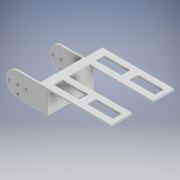
# Autodesk Inventor part: Claw
Saved by Autodesk Inventor 2020 (Build 240168000, 168)
## iProperties
Created: 2020-01-09
Part Number: Claw
Material: 일반
Document SubType Name: Modeling
Designer: Knowblesse
Density: 1 g/cm^3
Appearance: 기본값
Author: Knowblesse
Autodesk Inventor part; units mm, degrees
ref_plane "YZ Plane" through (0, 0, 0) normal (1, 0, 0) x (0, 1, 0)
ref_plane "XZ Plane" through (0, 0, 0) normal (0, 1, 0) x (-1, 0, 0)
ref_plane "XY Plane" through (0, 0, 0) normal (0, 0, 1) x (1, 0, 0)
sketch "스케치1" plane through (0, 0, 0) normal (0, 0, 1) x (1, 0, 0)
  line L0 (0, 0) -> (50, 0)
  line L1 (50, 0) -> (50, 28)
  line L2 (50, 28) -> (0, 28)
  line L3 (0, 28) -> (0, 0)
  circle A0 centre (14, 14) radius 14
  line L4 (0, 14) -> (50, 14) construction
  point P0 (14, 0)
  point P1 (14, 28)
  dimension "d0" = 36
  dimension "d1" = 28
  constraints: 10 end point, 2 midpoint, 2 parallel, 2 tangent, 1 centre point, 1 horizontal, 1 perpendicular, 1 point on line
  measures "d0" distance from line of L1 A0.centre
  measures "d1" diameter of A0
extrude "돌출1" add sketch "스케치1" along normal blind 54 contours A0 L2 L1 L0 | A0
sketch "스케치2" plane through (14, 28, 0) normal (0, 1, 0) x (1, 0, 0)
  line L0 (0, 0) -> (0, 0) projected
  line L1 (0, 0) -> (0, -54) projected
  line L2 (0, -54) -> (0, -54) projected
  line L3 (0, 0) -> (0, -54) projected
  line L4 (36, 0) -> (0, 0) projected
  line L5 (0, 0) -> (0, -54) projected
  line L6 (36, -54) -> (0, -54) projected
  line L7 (36, 0) -> (36, -54) projected
  line L8 (-14, -2) -> (25, -2)
  line L9 (25, -2) -> (25, -52)
  line L10 (25, -52) -> (-14, -52)
  line L11 (-14, -52) -> (-14, -2)
  line L12 (-14, 0) -> (0, 0) projected
  line L13 (36, 0) -> (36, -54) projected
  dimension "d4" = 2
  dimension "d5" = 2
  dimension "d6" = 11
  constraints: 8 end point, 2 parallel, 1 horizontal, 1 perpendicular, 1 vertical alignment
  measures "d4" distance between parallel lines of L4 L8
  measures "d5" distance between parallel lines of L6 L10
  measures "d6" distance between parallel lines of L13 L9
extrude "돌출2" cut sketch "스케치2" against normal up to surface (28 mm away) contours L8 L9 L10 L1 | L1 L10 L11 L8
sketch "스케치3" plane through (0, 0, 0) normal (0, 0, -1) x (-1, 0, 0)
  line L0 (-50, 0) -> (-50, 28) projected
  line L1 (-14, 0) -> (-50, 0) projected
  arc A0 (-14, 0) -> (-14, 28) centre (-14, 14) ccw projected
  line L2 (-50, 28) -> (-14, 28) projected
  point P0 (0, 0)
  point P1 (-14, 24)
  point P2 (-24, 14)
  point P3 (-14, 4)
  point P4 (-4, 14)
  dimension "d9" = 10
  dimension "d12" = 360
  constraints: 1 vertical alignment, 5 other
  measures "d9" distance of point (-14, 24) A0.centre
hole "구멍1" at (14, 24, 0) at (24, 14, 0) at (14, 4, 0) at (4, 14, 0) at (14, 14, 0) direction (0, 0, 1) diameter 3 end through all
sketch "스케치4" plane through (14, 28, 0) normal (0, 1, 0) x (1, 0, 0)
  line L0 (111, 21) -> (26, 21)
  line L1 (26, 21) -> (26, -4)
  line L2 (26, -4) -> (111, -4)
  line L3 (111, -4) -> (111, 21)
  line L4 (111, -29) -> (26, -29)
  line L5 (26, -29) -> (26, -54)
  line L6 (26, -54) -> (111, -54)
  line L7 (111, -54) -> (111, -29)
  line L8 (106, -36.5) -> (76, -36.5)
  line L9 (76, -36.5) -> (76, -46.5)
  line L10 (76, -46.5) -> (106, -46.5)
  line L11 (106, -46.5) -> (106, -36.5)
  line L12 (66, -36.5) -> (36, -36.5)
  line L13 (36, -36.5) -> (36, -46.5)
  line L14 (36, -46.5) -> (66, -46.5)
  line L15 (66, -46.5) -> (66, -36.5)
  line L16 (106, 13.5) -> (76, 13.5)
  line L17 (76, 13.5) -> (76, 3.5)
  line L18 (76, 3.5) -> (106, 3.5)
  line L19 (106, 3.5) -> (106, 13.5)
  line L20 (66, 13.5) -> (36, 13.5)
  line L21 (36, 13.5) -> (36, 3.5)
  line L22 (36, 3.5) -> (66, 3.5)
  line L23 (66, 3.5) -> (66, 13.5)
  line L24 (46, -4) -> (26, -4)
  line L25 (26, -4) -> (26, -29)
  line L26 (26, -29) -> (46, -29)
  line L27 (46, -29) -> (46, -4)
  line L28 (111, 8.5) -> (26, 8.5) construction
  line L29 (111, -41.5) -> (26, -41.5) construction
  line L30 (36, -54) -> (0, -54) construction
  line L31 (36, 0) -> (36, -54) construction
  point P0 (-14, 0)
  point P1 (106, 8.5)
  point P2 (106, -41.5)
  point P3 (66, -41.5)
  point P4 (66, 8.5)
  dimension "d21" = 25
  dimension "d22" = 25
  dimension "d23" = 25
  dimension "d24" = 10
  dimension "d25" = 10
  dimension "d26" = 30
  dimension "d27" = 30
  dimension "d28" = 10
  dimension "d29" = 10
  dimension "d30" = 5
  dimension "d31" = 10
  constraints: 60 end point, 14 parallel, 12 point on line, 8 midpoint, 7 horizontal, 7 perpendicular, 3 vertical alignment, 2 collinear
  measures "d21" distance between parallel lines of L0 L2
  measures "d22" distance between parallel lines of L6 L4
  measures "d23" distance between parallel lines of L4 L2
  measures "d24" distance between parallel lines of L18 L16
  measures "d25" distance of L10.end L8.start
  measures "d26" distance of L17.end L18.end
  measures "d27" distance of L21.end L22.end
  measures "d28" distance between parallel lines of L1 L21
  measures "d29" distance between parallel lines of L17 L23
  measures "d30" distance between parallel lines of L3 L19
  measures "d31" distance between parallel lines of L31 L27
extrude "돌출3" add sketch "스케치4" against normal blind 2 contours L3 L2 L1 L0 | L4 L7 L6 L5
